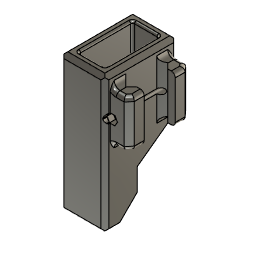
shell railed (Autodesk Fusion 360 archive; units mm, degrees)
design "rtlSDR mount"
Autodesk Fusion 360 part; units mm, degrees
sketch "Sketch1" plane through (0, 0, 0) normal (0, 0, 1) x (1, 0, 0)
  line L0 (0, 0) -> (13.3, 0)
  line L1 (13.3, 0) -> (13.3, 27.28)
  line L2 (13.3, 27.28) -> (0, 27.28)
  line L3 (0, 27.28) -> (0, 0)
  line L4 (0, 27.28) -> (13.3, 0)
  line L5 (18, 32) -> (-4.7, 32)
  line L6 (-4.7, 32) -> (-4.7, -4.72)
  line L7 (-4.7, -4.72) -> (18, -4.72)
  line L8 (18, -4.72) -> (18, 32)
  line L9 (18, 32) -> (-4.7, -4.72) construction
  line L10 (-4.7, 32) -> (18, -4.72) construction
  point P0 (6.65, 13.64)
  dimension "d1" = 13.3
  dimension "d2" = 27.28
  constraint horizontal L0
  constraint vertical L1
  constraint horizontal L2
  constraint vertical L3
  constraint coincident L0.start L3.end
  constraint horizontal L5
  constraint perpendicular L5 L6
  constraint parallel L5 L7
  constraint parallel L6 L8
  constraint coincident L9 P0
  constraint coincident L10 P0
  constraint midpoint L4 P0
  measures "d1" distance of L0.start L0.end
  measures "d2" distance of L0.start L2.end
extrude "Extrude1" add sketch "Sketch1" along normal blind 69
sketch "Sketch2" plane through (-4.7, 0, 0) normal (-1, 0, 0) x (0, -1, 0)
  line L0 (-32, 0) -> (4.72, 0)
  line L1 (4.72, 0) -> (4.72, 69)
  line L2 (4.72, 69) -> (-32, 69)
  line L3 (-32, 69) -> (-32, 0)
  line L4 (-13.64, 0) -> (-13.64, 21)
  line L5 (-13.64, 21) -> (-32, 34.5)
  constraint midpoint L0 L4.start
  constraint perpendicular L0 L4
  constraint midpoint L3 L5.end
extrude "Extrude2" cut sketch "Sketch2" against normal blind 53 contours L0 L3 L4 L5
chamfer "Chamfer1" distance 10 angle 45 2 edges at (15.65, 13.64, 0) (-2.35, 13.64, 0)
chamfer "Chamfer2" distance 2 angle 45 2 faces at (-4.7, 19.76, 57.5) (18, 19.76, 57.5)
chamfer "Chamfer3" distance 2 angle 45 2 edges at (6.65, 32, 69) (6.65, -4.72, 69)
fillet "Fillet1" radius 1 4 edges at (13.3, 0, 34.5) (0, 0, 34.5) (13.3, 27.28, 50.0147) (0, 27.28, 50.0147)
chamfer "Chamfer4" distance 2 angle 45 1 edges at (6.65, -4.72, 0)
fillet "Fillet2" radius 1 8 edges at (0.2929, 0.2929, 69) (0, 13.64, 69) (0.2929, 26.9871, 69) (6.65, 27.28, 69) (13.0071, 26.9871, 69) (13.3, 13.64, 69) (13.0071, 0.2929, 69) (6.65, 0, 69)
fillet "Fillet3" radius 1 14 edges at (13.3, 8.64, 5) (13.3, 2.32, 0) (13.0071, 0.2929, 0) (6.65, 0, 0) (0.2929, 0.2929, 0) (0, 2.32, 0) (0, 8.64, 5) (13.3, 13.64, 15.5) (0, 19.96, 25.6471) (0.2929, 26.9871, 30.814) (6.65, 27.28, 31.0294) (13.0071, 26.9871, 30.814) (13.3, 19.96, 25.6471) (0, 13.64, 15.5)
sketch "Sketch3" plane through (0, 32, 0) normal (0, 1, 0) x (-1, 0, 0)
  line L0 (2.7, 67) -> (-16, 67)
  line L1 (-16, 67) -> (-16, 34.5)
  line L2 (-16, 34.5) -> (2.7, 34.5)
  line L3 (2.7, 34.5) -> (2.7, 67)
  line L4 (2.7, 67) -> (-16, 67) construction
  line L5 (-16, 67) -> (-16, 34.5) construction
  line L6 (-16, 34.5) -> (2.7, 34.5) construction
  line L7 (2.7, 34.5) -> (2.7, 67) construction
  dimension "d17" = 6
  constraint coincident L0.end
  constraint coincident L2.end
sketch "Sketch4" plane through (0, 32, 0) normal (0, 1, 0) x (-1, 0, 0)
  line L0 (2.7, 67) -> (-16, 67)
  line L1 (-16, 67) -> (-16, 34.5)
  line L2 (-16, 34.5) -> (2.7, 34.5)
  line L3 (2.7, 34.5) -> (2.7, 67)
  line L4 (1, 60) -> (-14, 60) construction
  line L5 (-14, 60) -> (-14, 40) construction
  line L6 (-14, 40) -> (1, 40) construction
  line L7 (1, 40) -> (1, 60) construction
  dimension "d18" = 6
  text T0 "SDR" font "Calibri" height 6 align centre middle in box 15 x 20 at (1, 60) x (-1, 0) y (0, -1) spacing 1 kerned
extrude "Extrude3" cut sketch "Sketch4" against normal blind 1 text T0
sketch "Sketch5" plane through (0, 0, 69) normal (0, 0, 1) x (-1, 0, 0)
  line L0 (2.7, 2.72) -> (-16, 2.72)
  line L1 (-16, 2.72) -> (-16, -30)
  line L2 (-16, -30) -> (2.7, -30)
  line L3 (2.7, -30) -> (2.7, 2.72)
  arc A0 (1, -1) -> (-1, 1) centre (-1, -1) ccw
  line L4 (1, -1) -> (1, -26.28)
  arc A1 (-1, -28.28) -> (1, -26.28) centre (-1, -26.28) ccw
  line L5 (-1, -28.28) -> (-12.3, -28.28)
  arc A2 (-14.3, -26.28) -> (-12.3, -28.28) centre (-12.3, -26.28) ccw
  line L6 (-14.3, -26.28) -> (-14.3, -1)
  arc A3 (-12.3, 1) -> (-14.3, -1) centre (-12.3, -1) ccw
  line L7 (-12.3, 1) -> (-1, 1)
  line L8 (-14.3, -13.64) -> (-18, -13.64)
  line L9 (-18, -13.64) -> (-18, -21.475)
  line L10 (-18, -13.64) -> (-18, -5.805)
  line L11 (-18, -21.475) -> (-27.32, -21.475)
  line L12 (-18, -5.805) -> (-27.32, -5.805)
  line L13 (-18, -21.475) -> (-31.3987, -21.475) construction
  line L14 (-18, -5.805) -> (-30.8969, -5.805) construction
  line L15 (-18, -13.64) -> (-18, -24.24)
  line L16 (-18, -13.64) -> (-18, -3.04)
  line L17 (-18, -3.04) -> (-20.765, -3.04)
  line L18 (-18, -24.24) -> (-20.765, -24.24)
  line L19 (-20.765, -24.24) -> (-23.53, -21.475)
  line L20 (-20.765, -3.04) -> (-20.765, -6.6715)
  line L21 (-23.53, -21.475) -> (-23.53, -5.8047)
  line L22 (-20.765, -3.04) -> (-23.53, -5.8047)
  line L23 (-27.32, -5.805) -> (-27.32, -21.475)
  line L24 (-20.765, -24.24) -> (-18, -21.475)
  line L25 (-20.765, -3.04) -> (-18, -5.805)
  line L26 (-18, 2) -> (-25, 2)
  line L27 (-25, 2) -> (-25, -29)
  line L28 (-25, -29) -> (-18, -29)
  line L29 (-27.32, -21.475) -> (-27.32, -29)
  line L30 (-27.32, -5.805) -> (-27.32, 2)
  line L31 (-27.32, -21.475) -> (-27.32, -26.475)
  line L32 (-27.32, -5.805) -> (-27.32, -0.805)
  line L33 (-27.32, -26.475) -> (-25, -29)
  line L34 (-27.32, -0.805) -> (-25, 2)
  line L35 (-18, 2) -> (-18, -3.04)
  line L36 (-18, -29) -> (-18, -24.24)
  dimension "d21" = 7.835
  dimension "d22" = 7.835
  dimension "d23" = 9.32
  dimension "d24" = 9.32
  dimension "d27" = 10.6
  dimension "d28" = 10.6
  dimension "d29" = 45
  dimension "d30" = 45
  dimension "d31" = 5
  dimension "d32" = 5
  constraint midpoint L6 L8.start
  constraint perpendicular L1 L8
  constraint perpendicular L8 L9
  constraint perpendicular L8 L10
  constraint perpendicular L9 L11
  constraint perpendicular L10 L12
  constraint horizontal L13
  constraint horizontal L14
  constraint perpendicular L11 L15
  constraint perpendicular L8 L16
  constraint perpendicular L16 L17
  constraint perpendicular L15 L18
  constraint coincident L11 L19.end
  constraint vertical L21
  constraint perpendicular L19 L24
  constraint perpendicular L24 L25
  constraint perpendicular L23 L26
  constraint perpendicular L26 L27
  constraint perpendicular L27 L28
  constraint perpendicular L13 L29
  constraint perpendicular L14 L30
  constraint perpendicular L13 L31
  constraint perpendicular L14 L32
  constraint perpendicular L17 L35
  constraint perpendicular L18 L36
  measures "d21" distance of L8.end L9.end
  measures "d22" distance of L8.end L10.end
  measures "d23" distance of L9.end L11.end
  measures "d24" distance of L10.end L12.end
  measures "d27" distance of L8.end L15.end
  measures "d28" distance of L8.end L16.end
  measures "d29" angle of L18 L19
  measures "d30" angle of L19 L20
  measures "d31" distance of L11.end L31.end
  measures "d32" distance of L12.end L32.end
extrude "Extrude4" add sketch "Sketch5" against normal blind 30 contours L15 L18 L24 | L16 L17 L25 | L11 L18 L19 L27 L28 L36 | L12 L17 L22 L26 L27 L35 | L11 L27 L29 L31 L33 | L12 L27 L30 L32 L34
extrude "Extrude5" cut 2 faces at (21.255, 27.4133, 69) (21.255, -0.32, 69) along direction (0, 0, -1) blind 6.498
fillet "Fillet4" radius 3 2 edges at (18, 25.2375, 62.502) (18, 1.9025, 62.502)
fillet "Fillet5" radius 3 2 edges at (18, 25.2375, 39) (18, 1.9025, 39)
fillet "Fillet6" radius 2 8 edges at (27.32, 3.305, 39) (26.16, -0.5975, 39) (23, -2, 39) (18.8787, -2, 38.1213) (26.16, 27.7375, 39) (27.32, 23.975, 39) (18.8787, 29, 38.1213) (23, 29, 39)
fillet "Fillet7" radius 2 8 edges at (23, 29, 62.502) (18.8787, 29, 63.3807) (26.16, 27.7375, 62.502) (27.32, 23.975, 62.502) (18.8787, -2, 63.3807) (23, -2, 62.502) (26.16, -0.5975, 62.502) (27.32, 3.305, 62.502)
sketch "Sketch6" plane through (0, 32, 0) normal (0, 1, 0) x (-1, 0, 0)
  spline S0 degree 3 poles (-13.7023, 52.5431) (-13.7206, 52.59) (-13.7507, 52.6668) (-13.7756, 52.7455) (-13.7854, 52.7762) knots 0 0 0 0 0.015098 0.024749 0.024749 0.024749 0.024749
  spline S1 degree 3 poles (-13.7854, 52.7762) (-13.7907, 52.7958) (-13.8, 52.8299) (-13.8027, 52.8651) (-13.8038, 52.88) knots 0 0 0 0 0.006101 0.010568 0.010568 0.010568 0.010568
  spline S2 degree 3 poles (-13.8038, 52.88) (-13.8034, 52.8917) (-13.8025, 52.914) (-13.794, 52.9347) (-13.79, 52.9446) knots 0 0 0 0 0.003479 0.006653 0.006653 0.006653 0.006653
  spline S3 degree 3 poles (-13.79, 52.9446) (-13.7832, 52.9538) (-13.7677, 52.9747) (-13.7436, 52.985) (-13.73, 52.9908) knots 0 0 0 0 0.003354 0.007691 0.007691 0.007691 0.007691
  spline S4 degree 3 poles (-13.73, 52.9908) (-13.7117, 52.9967) (-13.6695, 53.0102) (-13.6256, 53.0155) (-13.6008, 53.0185) knots 0 0 0 0 0.005769 0.013243 0.013243 0.013243 0.013243
  spline S5 degree 3 poles (-13.6008, 53.0185) (-13.5685, 53.0211) (-13.4948, 53.0273) (-13.4208, 53.0275) (-13.3792, 53.0277) knots 0 0 0 0 0.009717 0.022181 0.022181 0.022181 0.022181
  spline S6 degree 3 poles (-13.3792, 53.0277) (-13.3429, 53.0275) (-13.2773, 53.0272) (-13.2121, 53.0211) (-13.1831, 53.0185) knots 0 0 0 0 0.010906 0.019645 0.019645 0.019645 0.019645
  spline S7 degree 3 poles (-13.1831, 53.0185) (-13.16, 53.0153) (-13.1181, 53.0097) (-13.0785, 52.995) (-13.0608, 52.9885) knots 0 0 0 0 0.006971 0.012627 0.012627 0.012627 0.012627
  spline S8 degree 3 poles (-13.0608, 52.9885) (-13.0464, 52.9811) (-13.0185, 52.9668) (-12.9988, 52.9425) (-12.9892, 52.9308) knots 0 0 0 0 0.004789 0.009279 0.009279 0.009279 0.009279
  spline S9 degree 3 poles (-12.9892, 52.9308) (-12.9809, 52.9171) (-12.963, 52.888) (-12.9515, 52.8557) (-12.9454, 52.8385) knots 0 0 0 0 0.00478 0.010244 0.010244 0.010244 0.010244
  line L0 (-12.9454, 52.8385) -> (-12.3962, 51.4308)
  spline S10 degree 3 poles (-12.3962, 51.4308) (-12.3642, 51.3536) (-12.3023, 51.2044) (-12.2302, 51.0598) (-12.1954, 50.99) knots 0 0 0 0 0.025044 0.048447 0.048447 0.048447 0.048447
  spline S11 degree 3 poles (-12.1954, 50.99) (-12.1598, 50.9261) (-12.0904, 50.8014) (-11.9949, 50.6954) (-11.9485, 50.6438) knots 0 0 0 0 0.021876 0.042641 0.042641 0.042641 0.042641
  spline S12 degree 3 poles (-11.9485, 50.6438) (-11.8984, 50.598) (-11.7976, 50.5055) (-11.6739, 50.4471) (-11.6115, 50.4177) knots 0 0 0 0 0.02024 0.040785 0.040785 0.040785 0.040785
  spline S13 degree 3 poles (-11.6115, 50.4177) (-11.541, 50.3942) (-11.3898, 50.3437) (-11.2304, 50.3393) (-11.1454, 50.3369) knots 0 0 0 0 0.022189 0.047539 0.047539 0.047539 0.047539
  line L1 (-11.1454, 50.3369) -> (-10.6146, 50.3369)
  line L2 (-10.6146, 50.3369) -> (-10.6146, 52.88)
  spline S14 degree 3 poles (-10.6146, 52.88) (-10.6138, 52.8918) (-10.6122, 52.9151) (-10.5999, 52.9349) (-10.5938, 52.9446) knots 0 0 0 0 0.0035 0.006881 0.006881 0.006881 0.006881
  spline S15 degree 3 poles (-10.5938, 52.9446) (-10.5855, 52.9535) (-10.5672, 52.9729) (-10.5426, 52.983) (-10.5292, 52.9885) knots 0 0 0 0 0.003633 0.00789 0.00789 0.00789 0.00789
  spline S16 degree 3 poles (-10.5292, 52.9885) (-10.512, 52.9938) (-10.4727, 53.0061) (-10.4321, 53.0125) (-10.4092, 53.0162) knots 0 0 0 0 0.005405 0.01233 0.01233 0.01233 0.01233
  spline S17 degree 3 poles (-10.4092, 53.0162) (-10.3806, 53.0195) (-10.317, 53.027) (-10.2529, 53.0274) (-10.2177, 53.0277) knots 0 0 0 0 0.00864 0.019201 0.019201 0.019201 0.019201
  spline S18 degree 3 poles (-10.2177, 53.0277) (-10.1825, 53.0274) (-10.1184, 53.027) (-10.0548, 53.0195) (-10.0262, 53.0162) knots 0 0 0 0 0.010562 0.019201 0.019201 0.019201 0.019201
  spline S19 degree 3 poles (-10.0262, 53.0162) (-10.0031, 53.0125) (-9.9618, 53.0059) (-9.9216, 52.9938) (-9.9038, 52.9885) knots 0 0 0 0 0.006982 0.012553 0.012553 0.012553 0.012553
  spline S20 degree 3 poles (-9.9038, 52.9885) (-9.89, 52.9832) (-9.865, 52.9736) (-9.8472, 52.9536) (-9.8392, 52.9446) knots 0 0 0 0 0.004361 0.00791 0.00791 0.00791 0.00791
  spline S21 degree 3 poles (-9.8392, 52.9446) (-9.8338, 52.9348) (-9.8228, 52.9147) (-9.8214, 52.8918) (-9.8208, 52.88) knots 0 0 0 0 0.003304 0.006796 0.006796 0.006796 0.006796
  line L3 (-9.8208, 52.88) -> (-9.8208, 47.3508)
  spline S22 degree 3 poles (-9.8208, 47.3508) (-9.8224, 47.2973) (-9.8254, 47.2017) (-9.8879, 47.1305) (-9.9154, 47.0992) knots 0 0 0 0 0.01547 0.027623 0.027623 0.027623 0.027623
  spline S23 degree 3 poles (-9.9154, 47.0992) (-9.9468, 47.0784) (-10.0079, 47.0379) (-10.0808, 47.031) (-10.1162, 47.0277) knots 0 0 0 0 0.011129 0.021609 0.021609 0.021609 0.021609
  line L4 (-10.1162, 47.0277) -> (-11.3854, 47.0277)
  spline S24 degree 3 poles (-11.3854, 47.0277) (-11.4544, 47.0279) (-11.5799, 47.0284) (-11.7052, 47.0359) (-11.7615, 47.0392) knots 0 0 0 0 0.020713 0.037639 0.037639 0.037639 0.037639
  spline S25 degree 3 poles (-11.7615, 47.0392) (-11.8091, 47.043) (-11.8992, 47.0502) (-11.9891, 47.06) (-12.0315, 47.0646) knots 0 0 0 0 0.014301 0.02712 0.02712 0.02712 0.02712
  spline S26 degree 3 poles (-12.0315, 47.0646) (-12.1414, 47.0865) (-12.3519, 47.1283) (-12.5489, 47.2133) (-12.6431, 47.2538) knots 0 0 0 0 0.0335 0.064173 0.064173 0.064173 0.064173
  spline S27 degree 3 poles (-12.6431, 47.2538) (-12.7272, 47.2989) (-12.8913, 47.387) (-13.0239, 47.5178) (-13.0885, 47.5815) knots 0 0 0 0 0.028465 0.05555 0.05555 0.05555 0.05555
  spline S28 degree 3 poles (-13.0885, 47.5815) (-13.1448, 47.6502) (-13.2577, 47.7881) (-13.3248, 47.9533) (-13.3585, 48.0362) knots 0 0 0 0 0.026481 0.053144 0.053144 0.053144 0.053144
  spline S29 degree 3 poles (-13.3585, 48.0362) (-13.3847, 48.1254) (-13.439, 48.3099) (-13.4452, 48.5022) (-13.4485, 48.6015) knots 0 0 0 0 0.027775 0.057457 0.057457 0.057457 0.057457
  spline S30 degree 3 poles (-13.4485, 48.6015) (-13.4457, 48.697) (-13.4406, 48.8795) (-13.3912, 49.0553) (-13.3677, 49.1392) knots 0 0 0 0 0.028514 0.054555 0.054555 0.054555 0.054555
  spline S31 degree 3 poles (-13.3677, 49.1392) (-13.3382, 49.2157) (-13.2799, 49.3665) (-13.1826, 49.4956) (-13.1346, 49.5592) knots 0 0 0 0 0.024462 0.048242 0.048242 0.048242 0.048242
  spline S32 degree 3 poles (-13.1346, 49.5592) (-13.0809, 49.6183) (-12.9718, 49.7381) (-12.8379, 49.8292) (-12.77, 49.8754) knots 0 0 0 0 0.023866 0.048409 0.048409 0.048409 0.048409
  spline S33 degree 3 poles (-12.77, 49.8754) (-12.696, 49.9187) (-12.544, 50.0075) (-12.3792, 50.0697) (-12.2946, 50.1015) knots 0 0 0 0 0.025665 0.052727 0.052727 0.052727 0.052727
  spline S34 degree 3 poles (-12.2946, 50.1015) (-12.3425, 50.1244) (-12.4375, 50.1696) (-12.5209, 50.2337) (-12.5623, 50.2654) knots 0 0 0 0 0.01587 0.031462 0.031462 0.031462 0.031462
  spline S35 degree 3 poles (-12.5623, 50.2654) (-12.6021, 50.3007) (-12.6838, 50.3732) (-12.7514, 50.459) (-12.7862, 50.5031) knots 0 0 0 0 0.015917 0.032708 0.032708 0.032708 0.032708
  spline S36 degree 3 poles (-12.7862, 50.5031) (-12.8208, 50.5521) (-12.893, 50.654) (-12.9518, 50.7643) (-12.9823, 50.8215) knots 0 0 0 0 0.017986 0.037436 0.037436 0.037436 0.037436
  spline S37 degree 3 poles (-12.9823, 50.8215) (-13.0137, 50.8851) (-13.0797, 51.0185) (-13.1369, 51.1558) (-13.1669, 51.2277) knots 0 0 0 0 0.021262 0.044624 0.044624 0.044624 0.044624
  line L5 (-13.1669, 51.2277) -> (-13.7023, 52.5431)
  spline S38 degree 3 poles (-7.8615, 47.8054) (-7.9756, 47.9392) (-8.2088, 48.2127) (-8.3425, 48.5465) (-8.4108, 48.7169) knots 0 0 0 0 0.052387 0.107054 0.107054 0.107054 0.107054
  spline S39 degree 3 poles (-8.4108, 48.7169) (-8.4653, 48.9057) (-8.5792, 49.3006) (-8.5914, 49.7116) (-8.5977, 49.9262) knots 0 0 0 0 0.058699 0.122792 0.122792 0.122792 0.122792
  spline S40 degree 3 poles (-8.5977, 49.9262) (-8.5916, 50.1699) (-8.5801, 50.6297) (-8.4571, 51.0726) (-8.3992, 51.2808) knots 0 0 0 0 0.072804 0.13737 0.13737 0.13737 0.13737
  spline S41 degree 3 poles (-8.3992, 51.2808) (-8.3277, 51.4633) (-8.1893, 51.8166) (-7.9403, 52.1025) (-7.82, 52.2408) knots 0 0 0 0 0.058314 0.112865 0.112865 0.112865 0.112865
  spline S42 degree 3 poles (-7.82, 52.2408) (-7.6839, 52.3604) (-7.4058, 52.6048) (-7.0613, 52.7411) (-6.8854, 52.8108) knots 0 0 0 0 0.053909 0.110204 0.110204 0.110204 0.110204
  spline S43 degree 3 poles (-6.8854, 52.8108) (-6.6842, 52.8659) (-6.2525, 52.9842) (-5.8046, 52.9945) (-5.5654, 53) knots 0 0 0 0 0.06233 0.133794 0.133794 0.133794 0.133794
  line L6 (-5.5654, 53) -> (-4.3008, 53)
  spline S44 degree 3 poles (-4.3008, 53) (-4.2654, 52.9967) (-4.1925, 52.9898) (-4.1315, 52.9493) (-4.1, 52.9285) knots 0 0 0 0 0.010481 0.021609 0.021609 0.021609 0.021609
  spline S45 degree 3 poles (-4.1, 52.9285) (-4.0725, 52.8971) (-4.01, 52.826) (-4.007, 52.7304) (-4.0054, 52.6769) knots 0 0 0 0 0.012152 0.027623 0.027623 0.027623 0.027623
  line L7 (-4.0054, 52.6769) -> (-4.0054, 47.3508)
  spline S46 degree 3 poles (-4.0054, 47.3508) (-4.007, 47.2973) (-4.01, 47.2017) (-4.0725, 47.1305) (-4.1, 47.0992) knots 0 0 0 0 0.01547 0.027623 0.027623 0.027623 0.027623
  spline S47 degree 3 poles (-4.1, 47.0992) (-4.1315, 47.0784) (-4.1925, 47.0379) (-4.2654, 47.031) (-4.3008, 47.0277) knots 0 0 0 0 0.011129 0.021609 0.021609 0.021609 0.021609
  line L8 (-4.3008, 47.0277) -> (-5.6531, 47.0277)
  spline S48 degree 3 poles (-5.6531, 47.0277) (-5.8933, 47.0331) (-6.3394, 47.0433) (-6.7667, 47.17) (-6.9638, 47.2285) knots 0 0 0 0 0.071714 0.133127 0.133127 0.133127 0.133127
  spline S49 degree 3 poles (-6.9638, 47.2285) (-7.1336, 47.3012) (-7.4653, 47.4432) (-7.7316, 47.6866) (-7.8615, 47.8054) knots 0 0 0 0 0.054956 0.107389 0.107389 0.107389 0.107389
  spline S50 degree 3 poles (-2.4431, 50.2562) (-2.5041, 50.3235) (-2.6279, 50.46) (-2.7105, 50.6249) (-2.7523, 50.7085) knots 0 0 0 0 0.027124 0.055019 0.055019 0.055019 0.055019
  spline S51 degree 3 poles (-2.7523, 50.7085) (-2.7866, 50.8023) (-2.8593, 51.0011) (-2.8663, 51.2128) (-2.87, 51.3246) knots 0 0 0 0 0.029781 0.063084 0.063084 0.063084 0.063084
  spline S52 degree 3 poles (-2.87, 51.3246) (-2.8646, 51.4585) (-2.8542, 51.7164) (-2.7605, 51.9567) (-2.7154, 52.0723) knots 0 0 0 0 0.03988 0.076824 0.076824 0.076824 0.076824
  spline S53 degree 3 poles (-2.7154, 52.0723) (-2.659, 52.1773) (-2.5467, 52.3864) (-2.3728, 52.548) (-2.2862, 52.6285) knots 0 0 0 0 0.035471 0.070683 0.070683 0.070683 0.070683
  spline S54 degree 3 poles (-2.2862, 52.6285) (-2.1893, 52.7003) (-1.9912, 52.8472) (-1.7588, 52.93) (-1.64, 52.9723) knots 0 0 0 0 0.03597 0.073555 0.073555 0.073555 0.073555
  spline S55 degree 3 poles (-1.64, 52.9723) (-1.512, 53.006) (-1.2496, 53.075) (-0.9783, 53.0834) (-0.8392, 53.0877) knots 0 0 0 0 0.039554 0.081135 0.081135 0.081135 0.081135
  spline S56 degree 3 poles (-0.8392, 53.0877) (-0.7427, 53.0859) (-0.556, 53.0824) (-0.3719, 53.0517) (-0.2831, 53.0369) knots 0 0 0 0 0.028932 0.055913 0.055913 0.055913 0.055913
  spline S57 degree 3 poles (-0.2831, 53.0369) (-0.2019, 53.0197) (-0.0471, 52.9869) (0.1027, 52.9363) (0.1738, 52.9123) knots 0 0 0 0 0.024882 0.047397 0.047397 0.047397 0.047397
  spline S58 degree 3 poles (0.1738, 52.9123) (0.236, 52.8887) (0.3514, 52.8448) (0.4605, 52.7868) (0.5108, 52.76) knots 0 0 0 0 0.019927 0.037007 0.037007 0.037007 0.037007
  spline S59 degree 3 poles (0.5108, 52.76) (0.5502, 52.7372) (0.6175, 52.6983) (0.6759, 52.6472) (0.7, 52.6262) knots 0 0 0 0 0.013637 0.023225 0.023225 0.023225 0.023225
  spline S60 degree 3 poles (0.7, 52.6262) (0.7167, 52.6059) (0.7514, 52.5638) (0.7692, 52.5122) (0.7785, 52.4854) knots 0 0 0 0 0.0078 0.016232 0.016232 0.016232 0.016232
  spline S61 degree 3 poles (0.7785, 52.4854) (0.7858, 52.4522) (0.8026, 52.3771) (0.8034, 52.3) (0.8038, 52.2569) knots 0 0 0 0 0.010161 0.023042 0.023042 0.023042 0.023042
  spline S62 degree 3 poles (0.8038, 52.2569) (0.8036, 52.2259) (0.8033, 52.1696) (0.7973, 52.1136) (0.7946, 52.0885) knots 0 0 0 0 0.009291 0.016881 0.016881 0.016881 0.016881
  spline S63 degree 3 poles (0.7946, 52.0885) (0.7915, 52.0681) (0.7859, 52.031) (0.7728, 51.9958) (0.7669, 51.98) knots 0 0 0 0 0.006167 0.01122 0.01122 0.01122 0.01122
  spline S64 degree 3 poles (0.7669, 51.98) (0.7609, 51.9675) (0.7499, 51.9447) (0.7298, 51.9293) (0.7208, 51.9223) knots 0 0 0 0 0.004086 0.007479 0.007479 0.007479 0.007479
  spline S65 degree 3 poles (0.7208, 51.9223) (0.7109, 51.9176) (0.6905, 51.9078) (0.6679, 51.9067) (0.6562, 51.9062) knots 0 0 0 0 0.003235 0.00672 0.00672 0.00672 0.00672
  spline S66 degree 3 poles (0.6562, 51.9062) (0.6297, 51.9114) (0.5636, 51.9244) (0.5075, 51.962) (0.4738, 51.9846) knots 0 0 0 0 0.008032 0.020018 0.020018 0.020018 0.020018
  spline S67 degree 3 poles (0.4738, 51.9846) (0.4294, 52.0125) (0.3313, 52.0742) (0.228, 52.1267) (0.1715, 52.1554) knots 0 0 0 0 0.015742 0.034736 0.034736 0.034736 0.034736
  spline S68 degree 3 poles (0.1715, 52.1554) (0.1042, 52.1865) (-0.0407, 52.2534) (-0.1926, 52.3023) (-0.2738, 52.3285) knots 0 0 0 0 0.022242 0.047822 0.047822 0.047822 0.047822
  spline S69 degree 3 poles (-0.2738, 52.3285) (-0.367, 52.352) (-0.5646, 52.4019) (-0.7685, 52.4067) (-0.8762, 52.4092) knots 0 0 0 0 0.028742 0.06094 0.06094 0.06094 0.06094
  spline S70 degree 3 poles (-0.8762, 52.4092) (-0.9591, 52.4068) (-1.1196, 52.402) (-1.2745, 52.3602) (-1.3492, 52.34) knots 0 0 0 0 0.02481 0.047958 0.047958 0.047958 0.047958
  spline S71 degree 3 poles (-1.3492, 52.34) (-1.4174, 52.3152) (-1.5497, 52.2671) (-1.6634, 52.1841) (-1.7185, 52.1438) knots 0 0 0 0 0.021644 0.041997 0.041997 0.041997 0.041997
  spline S72 degree 3 poles (-1.7185, 52.1438) (-1.7671, 52.099) (-1.8646, 52.0091) (-1.9256, 51.8914) (-1.9562, 51.8323) knots 0 0 0 0 0.019666 0.039454 0.039454 0.039454 0.039454
  spline S73 degree 3 poles (-1.9562, 51.8323) (-1.9804, 51.7672) (-2.0308, 51.6318) (-2.0363, 51.4874) (-2.0392, 51.4123) knots 0 0 0 0 0.020691 0.043057 0.043057 0.043057 0.043057
  spline S74 degree 3 poles (-2.0392, 51.4123) (-2.0354, 51.3323) (-2.028, 51.1792) (-1.9575, 51.0433) (-1.9238, 50.9785) knots 0 0 0 0 0.023714 0.045365 0.045365 0.045365 0.045365
  spline S75 degree 3 poles (-1.9238, 50.9785) (-1.8816, 50.9198) (-1.7953, 50.7998) (-1.6788, 50.7088) (-1.6192, 50.6623) knots 0 0 0 0 0.021561 0.044101 0.044101 0.044101 0.044101
  spline S76 degree 3 poles (-1.6192, 50.6623) (-1.5526, 50.6173) (-1.4147, 50.524) (-1.2651, 50.4509) (-1.1877, 50.4131) knots 0 0 0 0 0.024085 0.049888 0.049888 0.049888 0.049888
  spline S77 degree 3 poles (-1.1877, 50.4131) (-1.106, 50.375) (-0.9407, 50.2979) (-0.7752, 50.2211) (-0.6915, 50.1823) knots 0 0 0 0 0.02705 0.05472 0.05472 0.05472 0.05472
  spline S78 degree 3 poles (-0.6915, 50.1823) (-0.6075, 50.142) (-0.4395, 50.0615) (-0.2783, 49.9682) (-0.1977, 49.9215) knots 0 0 0 0 0.027942 0.055865 0.055865 0.055865 0.055865
  spline S79 degree 3 poles (-0.1977, 49.9215) (-0.1201, 49.872) (0.034, 49.7737) (0.166, 49.6473) (0.2315, 49.5846) knots 0 0 0 0 0.027556 0.054683 0.054683 0.054683 0.054683
  spline S80 degree 3 poles (0.2315, 49.5846) (0.2919, 49.5166) (0.4143, 49.3787) (0.4967, 49.2137) (0.5385, 49.13) knots 0 0 0 0 0.027148 0.055065 0.055065 0.055065 0.055065
  spline S81 degree 3 poles (0.5385, 49.13) (0.5728, 49.0354) (0.6459, 48.8335) (0.6526, 48.6187) (0.6562, 48.5046) knots 0 0 0 0 0.030001 0.063994 0.063994 0.063994 0.063994
  spline S82 degree 3 poles (0.6562, 48.5046) (0.6514, 48.3854) (0.6422, 48.1555) (0.5597, 47.9409) (0.52, 47.8377) knots 0 0 0 0 0.035529 0.068478 0.068478 0.068478 0.068478
  spline S83 degree 3 poles (0.52, 47.8377) (0.4705, 47.7442) (0.3724, 47.5588) (0.2181, 47.4166) (0.1415, 47.3462) knots 0 0 0 0 0.031473 0.06244 0.06244 0.06244 0.06244
  spline S84 degree 3 poles (0.1415, 47.3462) (0.0554, 47.2835) (-0.122, 47.1544) (-0.3289, 47.0814) (-0.4354, 47.0438) knots 0 0 0 0 0.031778 0.06544 0.06544 0.06544 0.06544
  spline S85 degree 3 poles (-0.4354, 47.0438) (-0.5507, 47.0136) (-0.7875, 46.9514) (-1.0322, 46.9439) (-1.1577, 46.94) knots 0 0 0 0 0.03565 0.073182 0.073182 0.073182 0.073182
  spline S86 degree 3 poles (-1.1577, 46.94) (-1.2242, 46.9415) (-1.358, 46.9445) (-1.4903, 46.9645) (-1.5569, 46.9746) knots 0 0 0 0 0.019923 0.04011 0.04011 0.04011 0.04011
  spline S87 degree 3 poles (-1.5569, 46.9746) (-1.6222, 46.9869) (-1.75, 47.0109) (-1.8745, 47.0485) (-1.9354, 47.0669) knots 0 0 0 0 0.019914 0.038981 0.038981 0.038981 0.038981
  spline S88 degree 3 poles (-1.9354, 47.0669) (-1.9918, 47.0861) (-2.0998, 47.1229) (-2.2025, 47.1725) (-2.2515, 47.1962) knots 0 0 0 0 0.017868 0.034183 0.034183 0.034183 0.034183
  spline S89 degree 3 poles (-2.2515, 47.1962) (-2.2908, 47.2162) (-2.3552, 47.2491) (-2.4117, 47.294) (-2.4338, 47.3115) knots 0 0 0 0 0.013174 0.02162 0.02162 0.02162 0.02162
  spline S90 degree 3 poles (-2.4338, 47.3115) (-2.4465, 47.3242) (-2.4678, 47.3455) (-2.4847, 47.3706) (-2.4915, 47.3808) knots 0 0 0 0 0.005348 0.00903 0.00903 0.00903 0.00903
  spline S91 degree 3 poles (-2.4915, 47.3808) (-2.4961, 47.3903) (-2.5059, 47.411) (-2.5116, 47.4333) (-2.5146, 47.4454) knots 0 0 0 0 0.003152 0.006876 0.006876 0.006876 0.006876
  spline S92 degree 3 poles (-2.5146, 47.4454) (-2.5176, 47.4598) (-2.5239, 47.491) (-2.5269, 47.5228) (-2.5285, 47.54) knots 0 0 0 0 0.004402 0.009569 0.009569 0.009569 0.009569
  spline S93 degree 3 poles (-2.5285, 47.54) (-2.5298, 47.5611) (-2.5328, 47.6088) (-2.533, 47.6565) (-2.5331, 47.6831) knots 0 0 0 0 0.006356 0.014318 0.014318 0.014318 0.014318
  spline S94 degree 3 poles (-2.5331, 47.6831) (-2.5329, 47.7092) (-2.5325, 47.7586) (-2.5282, 47.8077) (-2.5262, 47.8308) knots 0 0 0 0 0.007848 0.01479 0.01479 0.01479 0.01479
  spline S95 degree 3 poles (-2.5262, 47.8308) (-2.5238, 47.8507) (-2.5194, 47.8873) (-2.5098, 47.923) (-2.5054, 47.9392) knots 0 0 0 0 0.006005 0.011056 0.011056 0.011056 0.011056
  spline S96 degree 3 poles (-2.5054, 47.9392) (-2.5007, 47.9525) (-2.4922, 47.9769) (-2.4743, 47.9954) (-2.4662, 48.0038) knots 0 0 0 0 0.004159 0.007638 0.007638 0.007638 0.007638
  spline S97 degree 3 poles (-2.4662, 48.0038) (-2.4574, 48.0099) (-2.44, 48.022) (-2.419, 48.0237) (-2.4085, 48.0246) knots 0 0 0 0 0.003127 0.006229 0.006229 0.006229 0.006229
  spline S98 degree 3 poles (-2.4085, 48.0246) (-2.3864, 48.0202) (-2.3295, 48.0087) (-2.2797, 47.9785) (-2.2492, 47.96) knots 0 0 0 0 0.006716 0.017295 0.017295 0.017295 0.017295
  spline S99 degree 3 poles (-2.2492, 47.96) (-2.2092, 47.9368) (-2.1219, 47.8863) (-2.0323, 47.8398) (-1.9838, 47.8146) knots 0 0 0 0 0.013875 0.030263 0.030263 0.030263 0.030263
  spline S100 degree 3 poles (-1.9838, 47.8146) (-1.9272, 47.7877) (-1.8066, 47.7303) (-1.6796, 47.6889) (-1.6123, 47.6669) knots 0 0 0 0 0.018798 0.040018 0.040018 0.040018 0.040018
  spline S101 degree 3 poles (-1.6123, 47.6669) (-1.5367, 47.6474) (-1.3786, 47.6066) (-1.2153, 47.6023) (-1.13, 47.6) knots 0 0 0 0 0.023335 0.048832 0.048832 0.048832 0.048832
  spline S102 degree 3 poles (-1.13, 47.6) (-1.0517, 47.602) (-0.9042, 47.6059) (-0.7626, 47.6474) (-0.6962, 47.6669) knots 0 0 0 0 0.023368 0.044062 0.044062 0.044062 0.044062
  spline S103 degree 3 poles (-0.6962, 47.6669) (-0.6384, 47.6901) (-0.528, 47.7344) (-0.4356, 47.809) (-0.3915, 47.8446) knots 0 0 0 0 0.018559 0.035441 0.035441 0.035441 0.035441
  spline S104 degree 3 poles (-0.3915, 47.8446) (-0.354, 47.8833) (-0.279, 47.9607) (-0.234, 48.0587) (-0.2115, 48.1077) knots 0 0 0 0 0.016032 0.032084 0.032084 0.032084 0.032084
  spline S105 degree 3 poles (-0.2115, 48.1077) (-0.194, 48.1595) (-0.1587, 48.2644) (-0.1539, 48.3749) (-0.1515, 48.4308) knots 0 0 0 0 0.016325 0.033008 0.033008 0.033008 0.033008
  spline S106 degree 3 poles (-0.1515, 48.4308) (-0.1555, 48.5096) (-0.1632, 48.6612) (-0.2333, 48.7955) (-0.2669, 48.86) knots 0 0 0 0 0.023371 0.044916 0.044916 0.044916 0.044916
  spline S107 degree 3 poles (-0.2669, 48.86) (-0.3093, 48.9188) (-0.3964, 49.0396) (-0.5137, 49.1314) (-0.5738, 49.1785) knots 0 0 0 0 0.021642 0.044426 0.044426 0.044426 0.044426
  spline S108 degree 3 poles (-0.5738, 49.1785) (-0.6412, 49.2243) (-0.7806, 49.3191) (-0.9318, 49.3937) (-1.01, 49.4323) knots 0 0 0 0 0.024404 0.050519 0.050519 0.050519 0.050519
  spline S109 degree 3 poles (-1.01, 49.4323) (-1.0923, 49.471) (-1.2582, 49.5491) (-1.4246, 49.6264) (-1.5085, 49.6654) knots 0 0 0 0 0.02728 0.055026 0.055026 0.055026 0.055026
  spline S110 degree 3 poles (-1.5085, 49.6654) (-1.5928, 49.7056) (-1.7618, 49.7863) (-1.9251, 49.8779) (-2.0069, 49.9238) knots 0 0 0 0 0.02802 0.056162 0.056162 0.056162 0.056162
  spline S111 degree 3 poles (-2.0069, 49.9238) (-2.0859, 49.9725) (-2.2423, 50.0689) (-2.3766, 50.1942) (-2.4431, 50.2562) knots 0 0 0 0 0.027762 0.054952 0.054952 0.054952 0.054952
  line L9 (2.7, 67) -> (-16, 67)
  line L10 (-16, 67) -> (-16, 34.5)
  line L11 (-16, 34.5) -> (2.7, 34.5)
  line L12 (2.7, 34.5) -> (2.7, 67)
  circle A0 centre (-19, 50) radius 1.5
  circle A1 centre (-19, 50) radius 2.5
  dimension "d45" = 3
  dimension "d46" = 5
  constraint concentric A0 A1
  measures "d45" diameter of A0
  measures "d46" diameter of A1
extrude "Extrude6" cut sketch "Sketch6" against normal blind 3 contours A0 | A1
extrude "Extrude7" cut sketch "Sketch6" against normal blind 58 contours A0
extrude "Extrude8" cut sketch "Sketch6" along normal blind -42 and the other way blind 34 contours A1
sketch "Sketch7" plane through (0, -2, 0) normal (0, -1, 0) x (1, 0, 0)
  line L0 (18, 47.7087) -> (18, 40)
  arc A0 (21, 41) -> (18, 40) centre (21, 36) ccw
  line L1 (21, 41) -> (25, 41)
  line L2 (25, 41) -> (25, 60.502)
  line L3 (25, 60.502) -> (21, 60.502)
  arc A1 (18, 61.502) -> (21, 60.502) centre (21, 65.502) ccw
  line L4 (18, 61.502) -> (18, 52.2913)
  arc A2 (18, 52.2913) -> (18, 47.7087) centre (19, 50) ccw
  circle A3 centre (19, 50) radius 1.5
  line L5 (16.3737, 50.0564) -> (17.638, 47.7537)
  line L6 (17.638, 47.7537) -> (20.2644, 47.6973)
  line L7 (20.2644, 47.6973) -> (21.6263, 49.9436)
  line L8 (21.6263, 49.9436) -> (20.362, 52.2463)
  line L9 (20.362, 52.2463) -> (17.7356, 52.3027)
  line L10 (17.7356, 52.3027) -> (16.3737, 50.0564)
  point P0 (19, 50)
  dimension "d55" = 2.275
  constraint coincident P0 A2.centre
  measures "d55" distance of P0 L10
extrude "Extrude9" cut sketch "Sketch7" along normal blind 11.5 and the other way blind 3 contours A2 L5 L6 | L4 A2 L5 L6 L7 L8 L9 L10 | A2 L5 L10 | L4 A2 L9 L10
